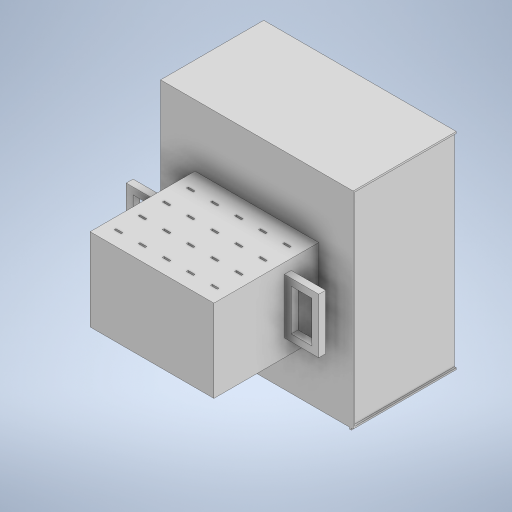
# Autodesk Inventor part: RP_Exterior
Saved by Autodesk Inventor 2024.3 (Build 283343000, 343)
## iProperties
Created: 2025-06-30
Part Number: RP_Exterior
Material: 一般
Document SubType Name: Modeling
Designer: 佐藤智貴
Density: 1 g/cm^3
Appearance: 既定
Mass: 3877.5 g
Surface Area: 14851 cm^2
Volume: 3877.5 cm^3
Author: 佐藤智貴
Autodesk Inventor part; units mm, degrees
ref_plane "YZ Plane" through (0, 0, 0) normal (1, 0, 0) x (0, 1, 0)
ref_plane "XZ Plane" through (0, 0, 0) normal (0, 1, 0) x (-1, 0, 0)
ref_plane "XY Plane" through (0, 0, 0) normal (0, 0, 1) x (1, 0, 0)
sketch "スケッチ1" plane through (0, 0, 0) normal (0, 0, 1) x (1, 0, 0)
  line L0 (0, 0) -> (350, 0)
  line L1 (350, 0) -> (350, 230)
  line L2 (350, 230) -> (0, 230)
  line L3 (0, 230) -> (0, 0)
  line L4 (-5, 235) -> (355, 235)
  line L5 (355, 235) -> (355, -5)
  line L6 (355, -5) -> (-5, -5)
  line L7 (-5, -5) -> (-5, 235)
  dimension "d0" = 350
  dimension "d1" = 230
  dimension "d2" = 5
  constraints: 16 end point, 4 parallel, 2 perpendicular, 1 horizontal, 3 other
  measures "d0" distance of L1.end L2.end
  measures "d1" distance of L0.end L1.end
  measures "d2" distance between parallel lines of L2 L4
extrude "押し出し1" add sketch "スケッチ1" along normal blind 300
sketch "スケッチ2" plane through (0, 0, 0) normal (0, 0, -1) x (-1, 0, 0)
  line L0 (-355, 235) -> (5, 235) projected
  line L1 (5, 235) -> (-355, 235)
  line L2 (-355, 235) -> (-355, 415)
  line L3 (-355, 415) -> (5, 415)
  line L4 (5, 415) -> (5, 235)
  line L5 (5, 415) -> (-355, 415)
  line L6 (-355, 415) -> (-355, -185)
  line L7 (-355, -185) -> (5, -185)
  line L8 (5, -185) -> (5, 415)
  line L9 (5, 235) -> (5, -5) projected
  line L10 (5, 115) -> (-355, 115)
  point P0 (0, 0)
  point P1 (-175, -185)
  dimension "d5" = 600
  dimension "d6" = 300
  dimension "d7" = 360
  constraints: 18 end point, 4 parallel, 3 midpoint, 3 perpendicular, 2 horizontal, 1 point on line
  measures "d5" distance between parallel lines of L7 L3
  measures "d6" distance from line of point (-175, -185) L10
  measures "d7" distance of L6.end L7.end
extrude "押し出し2" add sketch "スケッチ2" along normal blind 300
sketch "スケッチ3" plane through (0, 0, -300) normal (0, 0, -1) x (-1, 0, 0)
  line L0 (5, 415) -> (-355, 415) projected
  line L1 (-355, 415) -> (-355, -185) projected
  line L2 (-355, -185) -> (5, -185) projected
  line L3 (5, -185) -> (5, 415) projected
  line L4 (0, 410) -> (-350, 410)
  line L5 (-350, 410) -> (-350, -180)
  line L6 (-350, -180) -> (0, -180)
  line L7 (0, -180) -> (0, 410)
  point P0 (0, 0)
  dimension "d10" = 5
  constraints: 8 end point, 3 other
  measures "d10" distance between parallel lines of L3 L7
extrude "押し出し3" cut sketch "スケッチ3" against normal blind 295 contours L7 L6 L5 L4
sketch "スケッチ4" plane through (0, 0, 0) normal (0, 0, 1) x (1, 0, 0)
  line L0 (350, 230) -> (0, 230)
  line L1 (0, 230) -> (0, 0)
  line L2 (0, 0) -> (350, 0)
  line L3 (350, 0) -> (350, 230)
  constraints: 8 end point, 2 parallel, 1 horizontal, 1 perpendicular
extrude "押し出し4" cut sketch "スケッチ4" against normal blind 295
sketch "スケッチ5" plane through (-5, -5, 300) normal (-1, 0, 0) x (0, 0, 1)
  line L0 (-200, 210) -> (-220, 210)
  line L1 (-220, 210) -> (-220, 30)
  line L2 (-220, 30) -> (-200, 30)
  line L3 (-200, 30) -> (-200, 210)
  line L4 (-300, 240) -> (0, 240) projected
  line L5 (-300, 0) -> (0, 0) projected
  line L6 (0, 240) -> (0, 0) projected
  point P0 (-300, 5)
  dimension "d15" = 30
  dimension "d16" = 30
  dimension "d17" = 20
  dimension "d18" = 200
  constraints: 8 end point, 2 parallel, 1 horizontal, 1 perpendicular
  measures "d15" distance between parallel lines of L4 L0
  measures "d16" distance between parallel lines of L5 L2
  measures "d17" distance between parallel lines of L1 L3
  measures "d18" distance between parallel lines of L6 L3
extrude "押し出し5" add sketch "スケッチ5" along normal blind 100
sketch "スケッチ6" plane through (-5, 25, 100) normal (0, 0, 1) x (1, 0, 0)
  line L0 (0, 180) -> (0, 0) projected
  line L1 (0, 180) -> (-100, 180) projected
  line L2 (-100, 0) -> (-100, 180) projected
  line L3 (0, 0) -> (-100, 0) projected
  line L4 (-80, 160) -> (-20, 160)
  line L5 (-20, 160) -> (-20, 20)
  line L6 (-20, 20) -> (-80, 20)
  line L7 (-80, 20) -> (-80, 160)
  point P0 (5, -25)
  dimension "d21" = 20
  constraints: 8 end point, 3 other
  measures "d21" distance between parallel lines of L2 L7
extrude "押し出し6" cut sketch "スケッチ6" against normal blind 100 contours L4 L5 L6 L7
sketch "スケッチ8" plane through (355, -5, 300) normal (1, 0, 0) x (0, 0, -1)
  line L0 (200, 50) -> (220, 50) projected
  line L1 (200, 50) -> (220, 50)
  line L2 (220, 50) -> (220, 210)
  line L3 (220, 210) -> (200, 210)
  line L4 (200, 210) -> (200, 50)
  point P0 (300, 5)
  constraints: 8 end point, 2 parallel, 1 horizontal, 1 perpendicular
extrude "押し出し7" add sketch "スケッチ8" along normal blind 100
sketch "スケッチ9" plane through (355, 45, 100) normal (0, 0, 1) x (1, 0, 0)
  line L0 (0, 0) -> (0, 160) projected
  line L1 (0, 0) -> (100, 0) projected
  line L2 (100, 160) -> (100, 0) projected
  line L3 (0, 160) -> (100, 160) projected
  line L4 (80, 140) -> (80, 20)
  line L5 (80, 20) -> (20, 20)
  line L6 (20, 20) -> (20, 140)
  line L7 (20, 140) -> (80, 140)
  point P0 (-355, -45)
  point P1 (50, 140)
  dimension "d26" = 20
  constraints: 8 end point, 1 midpoint, 3 other
  measures "d26" distance from line of L3 point (50, 140)
extrude "押し出し8" cut sketch "スケッチ9" against normal blind 100 contours L4 L5 L6 L7
sketch "スケッチ10" plane through (355, -5, 300) normal (1, 0, 0) x (0, 0, -1)
  line L0 (305, -175) -> (305, 415) projected
  line L1 (600, -175) -> (600, 415) projected
  line L2 (305, -175) -> (600, -175)
  line L3 (600, -175) -> (600, 415)
  line L4 (600, 415) -> (305, 415)
  line L5 (305, 415) -> (305, -175)
  point P0 (300, 5)
  constraints: 8 end point, 2 parallel, 1 horizontal, 1 perpendicular
extrude "押し出し9" cut sketch "スケッチ10" against normal through all
sketch "スケッチ11" plane through (355, -5, 300) normal (1, 0, 0) x (0, 0, -1)
  line L0 (300, -180) -> (600, -180)
  line L1 (600, -180) -> (600, 420)
  line L2 (600, 420) -> (300, 420)
  line L3 (300, 420) -> (300, -180)
  line L4 (305, -175) -> (600, -175)
  line L5 (600, -175) -> (600, 415)
  line L6 (600, 415) -> (305, 415)
  line L7 (305, 415) -> (305, -175)
  point P0 (300, 5)
  dimension "d31" = 5
  constraints: 16 end point, 4 parallel, 2 horizontal, 2 perpendicular, 1 point on line
  measures "d31" distance between parallel lines of L2 L6
extrude "押し出し10" add sketch "スケッチ11" along normal blind 100 contours L3 L2 L1 L6 L7 L4 L0
sketch "スケッチ12" plane through (-5, -5, 300) normal (-1, 0, 0) x (0, 0, 1)
  line L0 (-300, 420) -> (-300, -180) projected
  line L1 (-300, -180) -> (-600, -180) projected
  line L2 (-300, 420) -> (-600, 420)
  line L3 (-600, 420) -> (-600, -180)
  line L4 (-600, -180) -> (-300, -180)
  line L5 (-300, -180) -> (-300, 420)
  line L6 (-600, 415) -> (-305, 415) projected
  line L7 (-305, 415) -> (-600, 415)
  line L8 (-600, 415) -> (-600, -175)
  line L9 (-600, -175) -> (-305, -175)
  line L10 (-305, -175) -> (-305, 415)
  point P0 (-300, 5)
  point P1 (-452.5, -175)
  dimension "d34" = 5
  constraints: 16 end point, 4 parallel, 2 horizontal, 2 perpendicular, 1 midpoint, 1 point on line
  measures "d34" distance from line of L1 point (-452.5, -175)
extrude "押し出し11" add sketch "スケッチ12" along normal blind 100 contours L0 L1 L3 L9 L10 L6 L2
sketch "スケッチ13" plane through (0, 0, 300) normal (0, 0, 1) x (1, 0, 0)
  line L0 (-5, -5) -> (355, -5) projected
  line L1 (355, 235) -> (-5, 235) projected
  line L2 (355, -5) -> (-5, -5)
  line L3 (-5, -5) -> (-5, 235)
  line L4 (-5, 235) -> (355, 235)
  line L5 (355, 235) -> (355, -5)
  point P0 (0, 0)
  constraints: 8 end point, 2 parallel, 1 horizontal, 1 perpendicular
extrude "押し出し12" add sketch "スケッチ13" along normal blind 5
sketch "スケッチ14" plane through (-5, 235, 0) normal (0, 1, 0) x (1, 0, 0)
  line L0 (330, -265) -> (310, -265)
  line L1 (310, -265) -> (310, -260)
  line L2 (310, -260) -> (330, -260)
  line L3 (330, -260) -> (330, -265)
  line L4 (360, -305) -> (0, -305) projected
  line L5 (360, 0) -> (360, -305) projected
  line L6 (260, -265) -> (240, -265)
  line L7 (260, -260) -> (260, -265)
  line L8 (240, -260) -> (260, -260)
  line L9 (240, -265) -> (240, -260)
  line L10 (190, -265) -> (170, -265)
  line L11 (190, -260) -> (190, -265)
  line L12 (170, -260) -> (190, -260)
  line L13 (170, -265) -> (170, -260)
  line L14 (120, -265) -> (100, -265)
  line L15 (120, -260) -> (120, -265)
  line L16 (100, -260) -> (120, -260)
  line L17 (100, -265) -> (100, -260)
  line L18 (50, -265) -> (30, -265)
  line L19 (50, -260) -> (50, -265)
  line L20 (30, -260) -> (50, -260)
  line L21 (30, -265) -> (30, -260)
  line L22 (0, 0) -> (0, -305) projected
  line L23 (190, -190) -> (190, -195)
  line L24 (190, -195) -> (170, -195)
  line L25 (170, -190) -> (190, -190)
  line L26 (170, -195) -> (170, -190)
  line L27 (120, -190) -> (120, -195)
  line L28 (120, -195) -> (100, -195)
  line L29 (100, -190) -> (120, -190)
  line L30 (100, -195) -> (100, -190)
  line L31 (50, -190) -> (50, -195)
  line L32 (30, -190) -> (50, -190)
  line L33 (50, -195) -> (30, -195)
  line L34 (30, -195) -> (30, -190)
  line L35 (240, -195) -> (240, -190)
  line L36 (260, -195) -> (240, -195)
  line L37 (240, -190) -> (260, -190)
  line L38 (260, -190) -> (260, -195)
  line L39 (310, -195) -> (310, -190)
  line L40 (330, -195) -> (310, -195)
  line L41 (310, -190) -> (330, -190)
  line L42 (330, -190) -> (330, -195)
  line L43 (190, -120) -> (190, -125)
  line L44 (190, -125) -> (170, -125)
  line L45 (170, -120) -> (190, -120)
  line L46 (170, -125) -> (170, -120)
  line L47 (120, -120) -> (120, -125)
  line L48 (120, -125) -> (100, -125)
  line L49 (100, -120) -> (120, -120)
  line L50 (100, -125) -> (100, -120)
  line L51 (50, -120) -> (50, -125)
  line L52 (30, -120) -> (50, -120)
  line L53 (50, -125) -> (30, -125)
  line L54 (30, -125) -> (30, -120)
  line L55 (240, -125) -> (240, -120)
  line L56 (260, -125) -> (240, -125)
  line L57 (240, -120) -> (260, -120)
  line L58 (260, -120) -> (260, -125)
  line L59 (310, -125) -> (310, -120)
  line L60 (330, -125) -> (310, -125)
  line L61 (310, -120) -> (330, -120)
  line L62 (330, -120) -> (330, -125)
  line L63 (190, -50) -> (190, -55)
  line L64 (190, -55) -> (170, -55)
  line L65 (170, -50) -> (190, -50)
  line L66 (170, -55) -> (170, -50)
  line L67 (120, -50) -> (120, -55)
  line L68 (120, -55) -> (100, -55)
  line L69 (100, -50) -> (120, -50)
  line L70 (100, -55) -> (100, -50)
  line L71 (50, -50) -> (50, -55)
  line L72 (30, -50) -> (50, -50)
  line L73 (50, -55) -> (30, -55)
  line L74 (30, -55) -> (30, -50)
  line L75 (240, -55) -> (240, -50)
  line L76 (260, -55) -> (240, -55)
  line L77 (240, -50) -> (260, -50)
  line L78 (260, -50) -> (260, -55)
  line L79 (310, -55) -> (310, -50)
  line L80 (330, -55) -> (310, -55)
  line L81 (310, -50) -> (330, -50)
  line L82 (330, -50) -> (330, -55)
  point P0 (5, 0)
  point P1 (320, -260)
  point P2 (250, -260)
  point P3 (180, -260)
  point P4 (110, -260)
  point P5 (40, -260)
  point P6 (30, -262.5)
  point P7 (30, -192.5)
  point P8 (180, -190)
  point P9 (110, -190)
  point P10 (40, -190)
  point P11 (250, -190)
  point P12 (320, -190)
  point P13 (30, -122.5)
  point P14 (180, -120)
  point P15 (110, -120)
  point P16 (40, -120)
  point P17 (250, -120)
  point P18 (320, -120)
  point P19 (30, -52.5)
  point P20 (180, -50)
  point P21 (110, -50)
  point P22 (40, -50)
  point P23 (250, -50)
  point P24 (320, -50)
  dimension "d39" = 20
  dimension "d40" = 5
  dimension "d41" = 40
  dimension "d42" = 30
  dimension "d45" = 70
  dimension "d50" = 30
  dimension "d53" = 70
  constraints: 160 end point, 2 horizontal, 2 midpoint, 2 parallel, 1 perpendicular, 1 vertical, 174 other
  measures "d39" distance of L0.start L0.end
  measures "d40" distance from line of point (320, -260) L0
  measures "d41" distance between parallel lines of L4 L0
  measures "d42" distance between parallel lines of L5 L3
  measures "d45" distance of L0.start L6.start
  measures "d50" distance from line of L22 point (30, -262.5)
  measures "d53" distance of point (30, -262.5) point (30, -192.5)
extrude "押し出し13" cut sketch "スケッチ14" against normal through all
sketch "スケッチ15" plane through (355, 410, -300) normal (0, -1, 0) x (1, 0, 0)
  line L0 (-360, 0) -> (-460, 0) projected
  line L1 (-460, 300) -> (-455, 300)
  line L2 (-455, 300) -> (-455, 0)
  line L3 (-455, 0) -> (-460, 0)
  line L4 (-460, 0) -> (-460, 300)
  line L5 (94.7122, 300) -> (89.7122, 300)
  line L6 (89.7122, 300) -> (89.7122, 0)
  line L7 (89.7122, 0) -> (94.7122, 0)
  line L8 (94.7122, 0) -> (94.7122, 300)
  point P0 (-355, 300)
  dimension "d60" = 5
  dimension "d61" = 5
  constraints: 16 end point, 4 parallel, 3 point on line, 2 horizontal, 2 perpendicular
  measures "d60" distance between parallel lines of L4 L2
  measures "d61" distance between parallel lines of L8 L6
extrude "押し出し14" add sketch "スケッチ15" along normal blind 600
equation "\"d6\" = 0.5 * d5"
equation "\"d16\" = d15"
